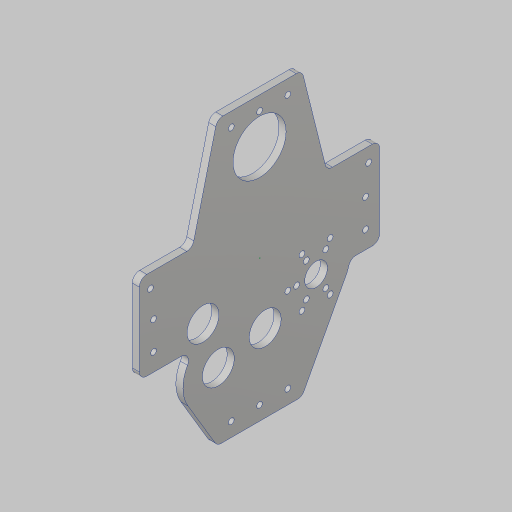
# Autodesk Inventor part: EL2-CGB-001
Saved by Autodesk Inventor 2023.5 (Build 275446000, 446)
## iProperties
Created: 2025-01-19
Part Number: EL2-CGB-001
Material: Aluminum 6061
Document SubType Name: Modeling
Designer: mavericks
Density: 2.7 g/cm^3
Appearance: Aluminum - Flat
Author: mavericks
Autodesk Inventor part; units mm, degrees
ref_plane "YZ Plane" through (0, 0, 0) normal (1, 0, 0) x (0, 1, 0)
ref_plane "XZ Plane" through (0, 0, 0) normal (0, 1, 0) x (-1, 0, 0)
ref_plane "XY Plane" through (0, 0, 0) normal (0, 0, 1) x (1, 0, 0)
sketch "Sketch1" plane through (0, 0, 0) normal (1, 0, 0) x (0, 1, 0)
  line L0 (127, 107.95) -> (-127, 107.95) construction
  line L1 (-127, 107.95) -> (-127, 82.55) construction
  line L2 (-127, 82.55) -> (127, 82.55) construction
  line L3 (127, 82.55) -> (127, 107.95) construction
  line L4 (-44.45, 128.7526) -> (-69.85, 128.7526) construction
  line L5 (-69.85, 128.7526) -> (-69.85, 79.4258) construction
  line L6 (-69.85, 79.4258) -> (-44.45, 79.4258) construction
  line L7 (-44.45, 79.4258) -> (-44.45, 128.7526) construction
  line L8 (69.85, 128.7526) -> (44.45, 128.7526) construction
  line L9 (44.45, 128.7526) -> (44.45, 79.4258) construction
  line L10 (44.45, 79.4258) -> (69.85, 79.4258) construction
  line L11 (69.85, 79.4258) -> (69.85, 128.7526) construction
  line L12 (44.45, 104.0892) -> (-44.45, 104.0892) construction
  line L13 (0, 0) -> (-27.2932, 0) construction
  line L14 (127, -107.95) -> (-127, -107.95) construction
  line L15 (-127, -107.95) -> (-127, -82.55) construction
  line L16 (-127, -82.55) -> (127, -82.55) construction
  line L17 (127, -82.55) -> (127, -107.95) construction
  line L18 (-44.45, -128.7526) -> (-69.85, -128.7526) construction
  line L19 (-69.85, -128.7526) -> (-69.85, -79.4258) construction
  line L20 (-69.85, -79.4258) -> (-44.45, -79.4258) construction
  line L21 (-44.45, -79.4258) -> (-44.45, -128.7526) construction
  line L22 (69.85, -128.7526) -> (44.45, -128.7526) construction
  line L23 (44.45, -128.7526) -> (44.45, -79.4258) construction
  line L24 (44.45, -79.4258) -> (69.85, -79.4258) construction
  line L25 (69.85, -79.4258) -> (69.85, -128.7526) construction
  line L26 (44.45, -104.0892) -> (-44.45, -104.0892) construction
  line L27 (127, 82.55) -> (101.6, 82.55) construction
  line L28 (101.6, 82.55) -> (101.6, -82.55) construction
  line L29 (101.6, -82.55) -> (127, -82.55) construction
  line L30 (127, -82.55) -> (127, 82.55) construction
  line L31 (-127, 82.55) -> (-101.6, 82.55) construction
  line L32 (-101.6, 82.55) -> (-101.6, -82.55) construction
  line L33 (-101.6, -82.55) -> (-127, -82.55) construction
  line L34 (-127, -82.55) -> (-127, 82.55) construction
  point P0 (0, 82.55)
  point P1 (0, 104.0892)
  point P2 (0, -82.55)
  point P3 (0, -104.0892)
  dimension "d0" = 254
  dimension "d1" = 25.4
  dimension "d2" = 82.55
  dimension "d3" = 25.4
  dimension "d4" = 49.3268
  dimension "d6" = 88.9
  dimension "d7" = 3.1242
  dimension "d8" = 25.4
  dimension "d9" = 25.4
  constraints: 70 end point, 16 symmetric about line, 12 parallel, 7 horizontal, 5 perpendicular, 4 midpoint, 2 vertical alignment, 1 horizontal alignment, 1 point on line
  measures "d0" distance of L2.end L1.end
  measures "d1" distance of L1.end L0.end
  measures "d2" vertical distance of L13.start L2.end
  measures "d3" distance of L6.end L5.end
  measures "d4" distance of L5.end L4.end
  measures "d6" distance of L4.start L8.end
  measures "d7" distance from line of L2 L6.end
  measures "d8" distance between parallel lines of L28 L30
  measures "d9" distance between parallel lines of L34 L32
sketch "Sketch2" plane through (0, 0, 0) normal (1, 0, 0) x (0, 1, 0)
  line L0 (-127, 107.95) -> (-127, 82.55) construction
  line L1 (44.45, 104.0892) -> (-44.45, 104.0892) construction
  line L2 (-127, 82.55) -> (127, 82.55) construction
  line L3 (127, 107.95) -> (-127, 107.95) construction
  line L4 (44.45, 79.4258) -> (69.85, 79.4258) construction
  line L5 (127, 82.55) -> (127, 107.95) construction
  line L6 (-69.85, 79.4258) -> (-44.45, 79.4258) construction
  line L7 (-44.45, 79.4258) -> (-44.45, 128.7526) construction
  line L8 (-69.85, 128.7526) -> (-69.85, 79.4258) construction
  line L9 (-44.45, 128.7526) -> (-69.85, 128.7526) construction
  line L10 (101.6, 82.55) -> (101.6, -82.55) construction
  line L11 (127, -82.55) -> (127, 82.55) construction
  line L12 (-127, -82.55) -> (127, -82.55) construction
  line L13 (127, -107.95) -> (-127, -107.95) construction
  line L14 (44.45, -104.0892) -> (-44.45, -104.0892) construction
  line L15 (-127, 82.55) -> (-101.6, 82.55) construction
  line L16 (-101.6, 82.55) -> (-101.6, -82.55) construction
  line L17 (-127, -82.55) -> (-127, 82.55) construction
  line L18 (-69.85, -79.4258) -> (-44.45, -79.4258) construction
  line L19 (-101.6, -82.55) -> (-127, -82.55) construction
  line L20 (-44.45, -79.4258) -> (-44.45, -128.7526) construction
  line L21 (-44.45, -128.7526) -> (-69.85, -128.7526) construction
  line L22 (-69.85, -128.7526) -> (-69.85, -79.4258) construction
  line L23 (-127, -107.95) -> (-127, -82.55) construction
  line L24 (44.45, -79.4258) -> (69.85, -79.4258) construction
  line L25 (44.45, -128.7526) -> (44.45, -79.4258) construction
  line L26 (101.6, -82.55) -> (127, -82.55) construction
  line L27 (69.85, -128.7526) -> (44.45, -128.7526) construction
  line L28 (69.85, -79.4258) -> (69.85, -128.7526) construction
  line L29 (127, -82.55) -> (127, -107.95) construction
  line L30 (69.85, 128.7526) -> (44.45, 128.7526) construction
  line L31 (44.45, 128.7526) -> (44.45, 79.4258) construction
  line L32 (69.85, 79.4258) -> (69.85, 128.7526) construction
  line L33 (127, 82.55) -> (101.6, 82.55) construction
  circle A0 centre (-38.1, -50.8) radius 7.62 construction
  circle A1 centre (-57.15, -5.08) radius 41.91 construction
  circle A2 centre (-57.15, -5.08) radius 11.43 construction
  circle A3 centre (-66.675, 37.0363) radius 31.75 construction
  circle A4 centre (-66.675, 37.0363) radius 15.24 construction
  circle A5 centre (-25.7473, 50.8) radius 27.94 construction
  circle A6 centre (-38.1, -50.8) radius 30.48 construction
  circle A7 centre (-38.1, -50.8) radius 10.16
  circle A8 centre (-57.15, -5.08) radius 14.2875
  circle A9 centre (-66.675, 37.0363) radius 14.2875
  circle A10 centre (-25.7473, 50.8) radius 14.2875
  circle A11 centre (-25.7473, 50.8) radius 20.6375 construction
  circle A12 centre (-66.675, 37.0363) radius 20.6375 construction
  circle A13 centre (-57.15, -5.08) radius 20.6375 construction
  circle A14 centre (-38.1, -50.8) radius 17.4625 construction
  circle A15 centre (-38.1, -50.8) radius 25.4 construction
  line L34 (-41.275, -131.9276) -> (-41.275, -76.2508) construction
  line L35 (-41.275, -76.2508) -> (-73.025, -76.2508) construction
  line L36 (-73.025, -76.2508) -> (-73.025, -131.9276) construction
  line L37 (-73.025, -131.9276) -> (-41.275, -131.9276) construction
  line L38 (-52.3959, -77.7195) -> (-127, -38.1)
  line L39 (-127, -38.1) -> (-127, 38.1)
  line L40 (-127, 38.1) -> (-41.275, 38.1) construction
  line L41 (-41.275, 38.1) -> (-41.275, 104.0892) construction
  arc A16 (-52.3959, -77.7195) -> (-41.275, -81.1142) centre (-38.1, -50.8) ccw
  circle A17 centre (86.4755, 0) radius 23.8125
  circle A18 centre (86.4755, 0) radius 33.3375 construction
  line L42 (37.9487, 60.325) -> (127, 38.1)
  line L43 (127, 38.1) -> (127, -38.1)
  line L44 (127, -38.1) -> (37.9487, -60.325)
  line L45 (37.9487, -60.325) -> (37.9487, -107.95)
  line L46 (37.9487, -107.95) -> (-41.275, -107.95)
  line L47 (-41.275, -107.95) -> (-41.275, -81.1142)
  line L48 (37.9487, 60.325) -> (37.9487, 107.95)
  line L49 (37.9487, 107.95) -> (-41.275, 107.95)
  arc A19 (-23.4758, 68.844) -> (-37.8063, 37.1865) centre (-25.7473, 50.8) ccw construction
  arc A20 (50.2903, -40.85) -> (93.2916, 54.1446) centre (86.4755, 0) ccw construction
  line L50 (-41.275, 107.95) -> (-41.275, 56.0863)
  line L51 (-82.9044, 64.325) -> (-127, 38.1)
  arc A21 (-41.275, 56.0863) -> (-82.9044, 64.325) centre (-66.675, 37.0363) ccw
  line L52 (93.2916, 54.1446) -> (-23.4758, 68.844) construction
  line L53 (50.2903, -40.85) -> (-37.8063, 37.1865) construction
  circle A22 centre (86.4755, 0) radius 11.1125 construction
  point P0 (25.2487, 98.0186)
  point P1 (0, 95.25)
  point P2 (25.2487, -98.0186)
  point P3 (0, -95.25)
  point P4 (-25.4, -95.25)
  point P5 (-25.4, 95.25)
  point P6 (127, -95.25)
  point P7 (127, 95.25)
  point P8 (0, -82.55)
  point P9 (-114.3, 25.4)
  point P10 (-114.3, 0)
  point P11 (-114.3, -25.4)
  point P12 (-101.6, 0)
  point P13 (-114.3, 82.55)
  point P14 (-38.1, -25.4)
  point P15 (-38.1, -33.3375)
  point P16 (-60.097, -38.1)
  point P17 (-53.223, -42.0688)
  point P18 (-60.097, -63.5)
  point P19 (-53.223, -59.5312)
  point P20 (-38.1, -76.2)
  point P21 (-38.1, -68.2625)
  point P22 (-16.103, -63.5)
  point P23 (-22.977, -59.5313)
  point P24 (-16.103, -38.1)
  point P25 (-22.977, -42.0688)
  point P26 (44.45, 104.0892)
  point P27 (-127, 0)
  point P28 (-127, 0)
  point P29 (101.6, 0)
  point P30 (114.3, 25.4)
  point P31 (114.3, 0)
  point P32 (114.3, -25.4)
  point P33 (114.3, 82.55)
  point P34 (127, 0)
  point P35 (-41.275, -76.8809)
  dimension "d33" = 34.925
  dimension "d34" = 50.8
  dimension "d10" = 15.24
  dimension "d11" = 83.82
  dimension "d12" = 22.86
  dimension "d13" = 63.5
  dimension "d14" = 30.48
  dimension "d15" = 55.88
  dimension "d16" = 60.96
  dimension "d19" = 63.5
  dimension "d23" = 20.32
  dimension "d24" = 28.575
  dimension "d26" = 25.4
  dimension "d27" = 25.4
  dimension "d28" = 25.4
  dimension "d29" = 25.4
  dimension "d30" = 6.35
  dimension "d31" = 6.35
  dimension "d32" = 6.35
  dimension "d37" = 360
  dimension "d41" = 3.175
  dimension "d42" = 76.2
  dimension "d60" = 101.7513
  dimension "d63" = 31.75
  dimension "d64" = 44.45
  dimension "d66" = 34.925
  dimension "d67" = 31.75
  dimension "d68" = 47.625
  dimension "d70" = 9.525
  dimension "d71" = 47.625
  dimension "d73" = 123.1853
  dimension "d74" = 12.7
  dimension "d75" = 36.3728
  dimension "d76" = 109.1438
  dimension "d78" = 9.9314
  dimension "d79" = 9.9314
  dimension "d133" = 204.1689
  dimension "d134" = 46.2281
  dimension "d135" = 117.689
  dimension "d141" = 22.225
  constraints: 40 end point, 21 centre point, 18 vertical alignment, 15 coincident, 12 point on circle, 11 horizontal alignment, 11 midpoint, 11 point on line, 9 tangent, 3 collinear, 2 equal radius, 2 perpendicular, 1 horizontal, 1 vertical, 20 other
  measures "d10" diameter of A0
  measures "d11" diameter of A1
  measures "d12" diameter of A2
  measures "d13" diameter of A3
  measures "d14" diameter of A4
  measures "d15" diameter of A5
  measures "d16" diameter of A6
  measures "d19" distance from line of L16 A0.centre
  measures "d23" diameter of A7
  measures "d24" diameter of A8
  measures "d26" distance of point (-25.4, 95.25) point (0, 95.25)
  measures "d27" distance of point (25.249, 98.019) point (0, 95.25)
  measures "d28" distance of point (-114.3, 0) point (-114.3, 25.4)
  measures "d29" distance of point (-114.3, 0) point (-114.3, -25.4)
  measures "d30" radial gap between concentric circles of A10 A11
  measures "d31" radial gap between concentric circles of A9 A12
  measures "d32" radial gap between concentric circles of A8 A13
  measures "d41" distance between parallel lines of L20 L34
  measures "d42" distance of L38.end L39.end
  measures "d60" distance from line of L5 point (25.249, 98.019)
  measures "d63" distance from line of L12 A0.centre
  measures "d64" distance from line of L16 A1.centre
  measures "d66" distance from line of L16 A3.centre
  measures "d67" distance from line of L2 A5.centre
  measures "d68" diameter of A17
  measures "d70" radial gap between concentric circles of A17 A18
  measures "d71" distance of L42.start L48.end
  measures "d73" distance of A17.centre A5.centre
  measures "d74" horizontal distance of point (25.249, 98.019) L48.end
  measures "d75" diameter of A19
  measures "d76" diameter of A20
  measures "d78" distance from line of point (25.249, 98.019) L3
  measures "d79" distance from line of L13 point (25.249, -98.019)
  measures "d135" distance of L52.start L52.end
  measures "d141" diameter of A22
extrude "Extrusion1" add sketch "Sketch2" along normal blind 6.35
hole "Mount Holes" at (0, -101.6, 82.55) at (0, -127, 107.95) at (0, -69.85, 79.4258) at (0, 44.45, -79.4258) at (0, 69.85, -79.4258) at (0, 44.45, -128.7526) at (0, 44.45, 128.7526) at (0, 25.2487, 98.0186) at (0, 0, 95.25) at (0, 25.2487, -98.0186) at (0, 0, -95.25) at (0, -25.4, -95.25) at (0, -25.4, 95.25) at (0, -114.3, 25.4) at (0, -114.3, 0) at (0, -114.3, -25.4) at (0, 114.3, 25.4) at (0, 114.3, 0) at (0, 114.3, -25.4) direction (1, 0, 0) diameter 5.1054 end through all clearance for "Flat Head Machine Screw (82)" size "#10" standard "Ansi Unified Screw Threads"
hole "Motor Mount Holes" at (0, -38.1, -33.3375) at (0, -60.097, -38.1) at (0, -53.223, -42.0688) at (0, -60.097, -63.5) at (0, -53.223, -59.5312) at (0, -16.103, -63.5) at (0, -22.977, -59.5313) at (0, -16.103, -38.1) at (0, -22.977, -42.0688) at (0, -38.1, -25.4) direction (1, 0, 0) diameter 5.1054 end through all clearance for "Flat Head Machine Screw (82)" size "#10" standard "Ansi Unified Screw Threads"
sketch "Sketch3" plane through (6.35, 0, 0) normal (1, 0, 0) x (0, 0, -1)
  point P0 (0, 0)
fillet "Fillet1" radius 6.604 12 edges at (3.175, -41.275, 107.95) (3.175, -127, 38.1) (3.175, -127, -38.1) (3.175, -41.275, -81.1142) (3.175, -41.275, -107.95) (3.175, 37.9487, -107.95) (3.175, 37.9487, -60.325) (3.175, 127, -38.1) (3.175, 127, 38.1) (3.175, 37.9487, 60.325) (3.175, 37.9487, 107.95) (3.175, -41.275, 56.0863)
sketch "Sketch4" plane through (6.35, 0, 0) normal (1, 0, 0) x (0, 0, -1)
  arc A0 (-107.95, -34.671) -> (-101.346, -41.275) centre (-101.346, -34.671) ccw construction
  line L0 (-107.95, -34.671) -> (-107.95, 31.3447) construction
  arc A1 (-101.346, 37.9487) -> (-107.95, 31.3447) centre (-101.346, 31.3447) ccw construction
  line L1 (-101.346, 37.9487) -> (-65.4834, 37.9487) construction
  arc A2 (-65.4834, 37.9487) -> (-59.0759, 42.9535) centre (-65.2807, 44.5527) ccw construction
  line L2 (-58.8844, 42.8978) -> (-39.4851, 109.5417) construction
  arc A3 (-33.1443, 114.3) -> (-39.4851, 109.5417) centre (-33.1443, 107.696) ccw construction
  line L3 (-33.1443, 114.3) -> (33.1443, 114.3) construction
  arc A4 (39.4851, 109.5417) -> (33.1443, 114.3) centre (33.1443, 107.696) ccw construction
  line L4 (39.4851, 109.5417) -> (58.9399, 42.7069) construction
  arc A5 (58.9399, 42.7069) -> (65.2807, 37.9487) centre (65.2807, 44.5527) ccw construction
  line L5 (65.2807, 37.9487) -> (101.346, 37.9487) construction
  arc A6 (107.95, 31.3447) -> (101.346, 37.9487) centre (101.346, 31.3447) ccw construction
  line L6 (107.95, 31.3447) -> (107.95, -34.671) construction
  arc A7 (101.346, -41.275) -> (107.95, -34.671) centre (101.346, -34.671) ccw construction
  line L7 (101.346, -41.275) -> (76.8809, -41.275) construction
  line L8 (76.8809, -41.275) -> (39.9622, -110.7934) construction
  arc A8 (34.1297, -114.3) -> (39.9622, -110.7934) centre (34.1297, -107.696) ccw construction
  line L9 (34.1297, -114.3) -> (-34.3439, -114.3) construction
  arc A9 (-40.02, -111.0717) -> (-34.3439, -114.3) centre (-34.3439, -107.696) ccw construction
  line L10 (-40.02, -111.0717) -> (-64.325, -70.2044) construction
  arc A10 (-68.3827, -48.9286) -> (-64.325, -70.2044) centre (-37.0363, -53.975) ccw construction
  arc A11 (-68.3827, -48.9286) -> (-74.9028, -41.275) centre (-74.9028, -47.879) ccw construction
  line L11 (-74.9028, -41.275) -> (-101.346, -41.275) construction
  circle A12 centre (38.1, -3.403) radius 2.5527 construction
  circle A13 centre (63.5, -3.403) radius 2.5527 construction
  circle A14 centre (63.5, -47.397) radius 2.5527 construction
  circle A15 centre (38.1, -47.397) radius 2.5527 construction
  circle A16 centre (33.3375, -25.4) radius 2.5527 construction
  circle A17 centre (42.0688, -40.523) radius 2.5527 construction
  circle A18 centre (59.5312, -40.523) radius 2.5527 construction
  circle A19 centre (59.5313, -10.277) radius 2.5527 construction
  circle A20 centre (42.0688, -10.277) radius 2.5527 construction
  circle A21 centre (0, 101.6) radius 2.5527 construction
  circle A22 centre (25.4, -101.6) radius 2.5527 construction
  circle A23 centre (-25.4, -101.6) radius 2.5527 construction
  circle A24 centre (95.25, -25.4) radius 2.5527 construction
  circle A25 centre (98.0186, 25.2487) radius 2.5527 construction
  circle A26 centre (-98.0186, 25.2487) radius 2.5527 construction
  circle A27 centre (-95.25, 0) radius 2.5527 construction
  circle A28 centre (95.25, 0) radius 2.5527 construction
  circle A29 centre (-95.25, -25.4) radius 2.5527 construction
  circle A30 centre (0, -101.6) radius 2.5527 construction
  circle A31 centre (-25.4, 101.6) radius 2.5527 construction
  circle A32 centre (25.4, 101.6) radius 2.5527 construction
  circle A33 centre (0, 58.3056) radius 23.8125 construction
  circle A34 centre (-50.8, -13.0473) radius 14.2875 construction
  circle A35 centre (-37.0363, -53.975) radius 14.2875 construction
  circle A36 centre (5.08, -44.45) radius 14.2875 construction
  circle A37 centre (50.8, -25.4) radius 10.16 construction
  circle A38 centre (0, 58.3056) radius 30.1625 construction
  circle A39 centre (-50.8, -13.0473) radius 20.6375 construction
  circle A40 centre (-37.0363, -53.975) radius 20.6375 construction
  circle A41 centre (5.08, -44.45) radius 20.6375 construction
  circle A42 centre (38.1, -3.403) radius 8.9027 construction
  circle A43 centre (63.5, -3.403) radius 8.9027 construction
  line L12 (0, 58.3056) -> (-50.8, -13.0473) construction
  circle A44 centre (63.5, -16.103) radius 2.5527 construction
  line L13 (0, 58.3056) -> (69.8474, -9.5713) construction
  line L14 (0, 58.3056) -> (5.08, -44.45) construction
  line L15 (-47.1323, -13.3701) -> (0.4406, 53.4502) construction
  line L16 (0.4406, 53.4502) -> (74.8023, -18.8136) construction
  line L17 (-52.3052, -9.6872) -> (-0.4406, 63.1611) construction
  line L18 (-0.4406, 63.1611) -> (79.2277, -14.2597) construction
  line L19 (8.3838, -46.9773) -> (3.5692, 50.4098) construction
  line L20 (3.5692, 50.4098) -> (74.8023, -18.8136) construction
  line L21 (2.0416, -47.2908) -> (-3.5692, 66.2014) construction
  line L22 (-3.5692, 66.2014) -> (79.2277, -14.2597) construction
  line L23 (-65.2807, 31.5987) -> (-101.346, 31.5987) construction
  arc A45 (-101.346, 31.5987) -> (-101.6, 31.3447) centre (-101.346, 31.3447) ccw construction
  line L24 (-101.6, 31.3447) -> (-101.6, -34.671) construction
  arc A46 (-101.6, -34.671) -> (-101.346, -34.925) centre (-101.346, -34.671) ccw construction
  line L25 (-101.346, -34.925) -> (-74.9028, -34.925) construction
  arc A47 (-62.1135, -49.9379) -> (-74.9028, -34.925) centre (-74.9028, -47.879) ccw construction
  arc A48 (-62.1135, -49.9379) -> (-58.8673, -66.9585) centre (-37.0363, -53.975) ccw construction
  line L26 (-58.8673, -66.9585) -> (-34.5622, -107.8258) construction
  arc A49 (-34.5622, -107.8258) -> (-34.3439, -107.95) centre (-34.3439, -107.696) ccw construction
  line L27 (-34.3439, -107.95) -> (34.1297, -107.95) construction
  arc A50 (34.1297, -107.95) -> (34.354, -107.8151) centre (34.1297, -107.696) ccw construction
  line L28 (34.354, -107.8151) -> (71.2726, -38.2967) construction
  arc A51 (71.2726, -38.2967) -> (62.2649, -29.6267) centre (44.45, -57.15) ccw construction
  arc A52 (58.1608, -34.925) -> (62.2649, -29.6267) centre (80.3564, -47.879) ccw construction
  line L29 (58.1608, -34.925) -> (101.346, -34.925) construction
  arc A53 (101.346, -34.925) -> (101.0948, -34.7088) centre (101.346, -34.671) ccw construction
  line L30 (101.6, -34.925) -> (101.6, 31.3447) construction
  arc A54 (101.6, 31.3447) -> (101.346, 31.5987) centre (101.346, 31.3447) ccw construction
  line L31 (101.346, 31.5987) -> (65.2807, 31.5987) construction
  arc A55 (52.843, 40.9322) -> (65.2807, 31.5987) centre (65.2807, 44.5527) ccw construction
  line L32 (52.843, 40.9322) -> (33.3881, 107.767) construction
  arc A56 (33.3881, 107.767) -> (33.1443, 107.95) centre (33.1443, 107.696) ccw construction
  line L33 (33.1443, 107.95) -> (-33.1443, 107.95) construction
  arc A57 (-33.1443, 107.95) -> (-33.3881, 107.767) centre (-33.1443, 107.696) ccw construction
  line L34 (-33.3881, 107.767) -> (-52.843, 40.9322) construction
  arc A58 (-65.2807, 31.5987) -> (-52.843, 40.9322) centre (-65.2807, 44.5527) ccw construction
  circle A59 centre (0, -114.3) radius 2.5527 construction
  circle A60 centre (38.1, -60.097) radius 2.5527 construction
  circle A61 centre (38.1, -47.397) radius 8.9027 construction
  circle A62 centre (-25.4, -101.6) radius 8.9027 construction
  circle A63 centre (25.4, -101.6) radius 8.9027 construction
  line L35 (-14.81, 32.0294) -> (-36.3867, 1.723)
  line L36 (19.2982, 35.1246) -> (55.3225, 0.1166)
  line L37 (-31.239, -6.4691) -> (-25.4065, -23.8125)
  line L38 (40.9805, 5.0209) -> (55.3225, 0.1166)
  line L39 (-25.4065, -23.8125) -> (0.8809, -23.8125)
  arc A64 (-31.239, -6.4691) -> (-36.3867, 1.723) centre (-50.8, -13.0473) ccw
  arc A65 (40.9805, 5.0209) -> (32.5805, 3.5823) centre (38.1, -3.403) ccw
  arc A66 (-14.81, 32.0294) -> (19.2982, 35.1246) centre (0, 58.3056) ccw
  line L40 (6.8879, -16.719) -> (4.6522, 28.5041)
  line L41 (-1.6901, 28.1905) -> (0.8809, -23.8125)
  line L42 (6.8879, -16.719) -> (32.5805, 3.5823)
  line L43 (59.9983, 0) -> (57.5056, 34.1915) construction
  circle A67 centre (95.25, -25.4) radius 2.5527 construction
  line L44 (59.9983, 0) -> (95.25, 0) construction
  line L45 (60.8203, 32.3908) -> (62.9502, 3.175) construction
  line L46 (62.9502, 3.175) -> (95.5186, 3.175) construction
  line L47 (54.0356, 38.122) -> (57.0463, -3.175) construction
  line L48 (57.0463, -3.175) -> (95.25, -3.175) construction
  circle A68 centre (95.25, -25.4) radius 8.9027 construction
  circle A69 centre (95.25, 0) radius 8.9027 construction
  circle A70 centre (98.0186, 25.2487) radius 8.9027 construction
  circle A71 centre (98.0186, 25.2487) radius 2.5527 construction
  arc A72 (91.7788, 31.5987) -> (101.6, 17.0981) centre (98.0186, 25.2487) ccw
  circle A73 centre (95.25, 0) radius 2.5527 construction
  arc A74 (101.6, 6.2398) -> (86.9327, 3.175) centre (95.25, 0) ccw
  arc A75 (86.9327, -3.175) -> (101.6, -6.2398) centre (95.25, 0) ccw
  arc A76 (101.6, -19.1602) -> (88.9, -31.6398) centre (95.25, -25.4) ccw
  line L49 (61.9926, -15.9214) -> (60.0394, -32.1415) construction
  line L50 (63.6988, -28.3093) -> (66.8402, -2.2217) construction
  line L51 (66.8402, -2.2217) -> (-3.5692, 66.2014) construction
  line L52 (-3.5692, 66.2014) -> (2.0416, -47.2908) construction
  line L53 (57.7912, -24.2546) -> (60.1598, -4.5842) construction
  line L54 (60.1598, -4.5842) -> (3.5692, 50.4098) construction
  line L55 (3.5692, 50.4098) -> (8.3838, -46.9773) construction
  line L56 (60.8203, 32.3908) -> (62.9502, 3.175)
  line L57 (62.9502, 3.175) -> (86.9327, 3.175)
  line L58 (86.9327, -3.175) -> (67.8212, -3.175)
  line L59 (67.8212, -3.175) -> (59.748, 4.6705)
  arc A77 (65.6579, -12.0402) -> (59.748, 4.6705) centre (63.5, -3.403) ccw
  arc A78 (58.1608, -34.925) -> (63.6988, -28.3093) centre (80.3564, -47.879) ccw
  line L60 (58.1608, -34.925) -> (88.9, -34.925)
  line L61 (63.6988, -28.3093) -> (65.6579, -12.0402)
  line L62 (91.7788, 31.5987) -> (65.2807, 31.5987)
  arc A79 (60.8203, 32.3908) -> (65.2807, 31.5987) centre (65.2807, 44.5527) ccw
  line L63 (101.6, 17.0981) -> (101.6, 6.2398)
  line L64 (29.4865, 51.9556) -> (49.6342, 51.9556)
  arc A80 (23.7236, 39.6786) -> (29.4865, 51.9556) centre (0, 58.3056) ccw
  arc A81 (52.843, 40.9322) -> (54.0356, 38.122) centre (65.2807, 44.5527) ccw
  line L65 (49.6342, 51.9556) -> (52.843, 40.9322)
  line L66 (54.0356, 38.122) -> (56.2247, 8.0943)
  line L67 (56.2247, 8.0943) -> (23.7236, 39.6786)
  line L68 (-29.4865, 51.9556) -> (-49.6342, 51.9556)
  line L69 (-50.8, -13.0473) -> (-57.5056, 34.1915) construction
  line L70 (-47.6565, -12.6011) -> (-54.7072, 37.0689) construction
  line L71 (-53.9435, -13.4936) -> (-60.1282, 30.0756) construction
  circle A82 centre (-95.25, 0) radius 8.9027 construction
  circle A83 centre (-98.0186, 25.2487) radius 8.9027 construction
  circle A84 centre (-95.25, -25.4) radius 8.9027 construction
  circle A85 centre (-95.25, 0) radius 2.5527 construction
  line L72 (-95.25, 0) -> (-66.7898, 0) construction
  line L73 (-95.25, 3.175) -> (-63.5571, 3.175) construction
  line L74 (-95.25, -3.175) -> (-69.223, -3.175) construction
  line L75 (-65.2807, 31.5987) -> (-91.7788, 31.5987)
  line L76 (-101.6, 17.0981) -> (-101.6, 6.2398)
  line L77 (-101.6, -6.2398) -> (-101.6, -19.1602)
  line L78 (-88.9, -34.925) -> (-74.9028, -34.925)
  line L79 (-62.1135, -49.9379) -> (-57.2751, -49.9379)
  line L80 (-86.9327, 3.175) -> (-63.5571, 3.175)
  line L81 (-68.923, -3.175) -> (-86.9327, -3.175)
  line L82 (-60.4755, 32.5229) -> (-56.8094, 6.6959)
  line L83 (-50.5224, 7.5883) -> (-54.7072, 37.0689)
  line L84 (-41.5596, 5.4059) -> (-19.9829, 35.7123)
  circle A86 centre (-98.0186, 25.2487) radius 2.5527 construction
  arc A87 (-101.6, 17.0981) -> (-91.7788, 31.5987) centre (-98.0186, 25.2487) ccw
  arc A88 (-86.9327, 3.175) -> (-101.6, 6.2398) centre (-95.25, 0) ccw
  arc A89 (-101.6, -6.2398) -> (-86.9327, -3.175) centre (-95.25, 0) ccw
  arc A90 (-88.9, -31.6398) -> (-101.6, -19.1602) centre (-95.25, -25.4) ccw
  arc A91 (-62.1135, -49.9379) -> (-74.9028, -34.925) centre (-74.9028, -47.879) ccw
  arc A92 (-49.7363, -37.708) -> (-57.2751, -49.9379) centre (-37.0363, -53.975) ccw
  line L85 (-49.7363, -37.708) -> (-49.7363, -33.6574)
  arc A93 (-68.923, -3.175) -> (-49.7363, -33.6574) centre (-50.8, -13.0473) ccw
  arc A94 (-56.8094, 6.6959) -> (-63.5571, 3.175) centre (-50.8, -13.0473) ccw
  arc A95 (-65.4834, 37.9487) -> (-59.0759, 42.9535) centre (-65.4834, 44.5527) ccw construction
  arc A96 (-65.2807, 31.5987) -> (-60.4755, 32.5229) centre (-65.2807, 44.5527) ccw
  arc A97 (-29.4865, 51.9556) -> (-19.9829, 35.7123) centre (0, 58.3056) ccw
  line L86 (-49.6342, 51.9556) -> (-52.843, 40.9322)
  arc A98 (-54.7072, 37.0689) -> (-52.843, 40.9322) centre (-65.2807, 44.5527) ccw
  line L87 (-43.3863, -73.6113) -> (-49.5945, -82.55)
  line L88 (-25.4, -92.6973) -> (25.4, -92.6973)
  line L89 (25.4, -92.6973) -> (29.2279, -46.6594)
  line L90 (29.2325, -46.6056) -> (25.6358, -46.2846)
  line L91 (-11.187, -57.15) -> (-16.6445, -57.15)
  line L92 (-49.5945, -82.55) -> (-34.4884, -107.95)
  line L93 (-34.4884, -107.95) -> (-31.6398, -107.95)
  arc A99 (-43.3863, -73.6113) -> (-16.6445, -57.15) centre (-37.0363, -53.975) ccw
  arc A100 (-11.187, -57.15) -> (25.6358, -46.2846) centre (5.08, -44.45) ccw
  arc A101 (29.2325, -46.6056) -> (29.2279, -46.6594) centre (38.1, -47.397) ccw
  circle A102 centre (-25.4, -114.3) radius 2.5527 construction
  arc A103 (-25.4, -92.6973) -> (-31.6398, -107.95) centre (-25.4, -101.6) ccw
  arc A104 (-41.5596, 5.4059) -> (-50.5224, 7.5883) centre (-50.8, -13.0473) ccw
  line L94 (101.6, -19.1602) -> (101.6, -6.2398)
  line L95 (-88.9, -31.6398) -> (-88.9, -34.925)
  line L96 (88.9, -34.925) -> (88.9, -31.6398)
  circle A105 centre (25.4, -25.4) radius 2.5527 projected
  point P0 (0, 0)
  point P1 (60.0394, -32.1415)
  point P2 (31.75, 27.4513)
  point P3 (-49.7363, -35.6827)
  point P4 (-42.0415, -95.25)
  point P5 (-51.5708, -29.9236)
  point P6 (30.5287, -26.3344)
  point P7 (-101.6, 6.2398)
  point P8 (-88.9, -33.2824)
  point P9 (88.9, -33.2824)
  point P10 (72.3998, -3.175)
  point P11 (86.685, -22.9712)
  dimension "d80" = 6.35
  dimension "d81" = 6.35
  dimension "d82" = 6.35
  dimension "d83" = 6.35
  dimension "d84" = 6.35
  dimension "d85" = 6.35
  dimension "d86" = 3.175
  dimension "d87" = 3.175
  dimension "d88" = 3.175
  dimension "d89" = 3.175
  dimension "d90" = 6.35
  dimension "d91" = 6.35
  dimension "d94" = 6.35
  dimension "d95" = 6.35
  dimension "d96" = 3.175
  dimension "d97" = 3.175
  dimension "d98" = 6.35
  dimension "d99" = 6.35
  dimension "d100" = 6.35
  dimension "d101" = 3.175
  dimension "d102" = 3.175
  dimension "d103" = 3.175
  dimension "d104" = 3.175
  dimension "d105" = 3.175
  dimension "d106" = 6.35
  dimension "d107" = 3.175
  dimension "d108" = 3.175
  dimension "d109" = 6.35
  dimension "d110" = 6.35
  dimension "d111" = 6.35
  dimension "d112" = 3.175
  dimension "d113" = 3.175
  dimension "d114" = 12.7
  dimension "d115" = 6.35
  dimension "d116" = 31.75
  dimension "d117" = 12.7
  dimension "d121" = 12.7
  dimension "d122" = 12.7
  constraints: 169 end point, 129 point on circle, 53 centre point, 39 point on line, 23 coincident, 9 horizontal, 8 collinear, 8 tangent, 5 parallel, 4 horizontal alignment, 4 midpoint, 4 vertical alignment, 3 vertical, 2 concentric, 2 line through centre, 56 other
  measures "d80" radial gap between concentric circles of A33 A38
  measures "d82" radial gap between concentric circles of A35 A40
  measures "d83" radial gap between concentric circles of A36 A41
  measures "d84" radial gap between concentric circles of A12 A42
  measures "d85" radial gap between concentric circles of A13 A43
  measures "d86" distance between parallel lines of L12 L15
  measures "d87" distance between parallel lines of L12 L17
  measures "d88" distance between parallel lines of L14 L19
  measures "d89" distance between parallel lines of L14 L21
  measures "d90" distance between parallel lines of L1 L23
  measures "d91" radial gap between concentric circles of A15 A61
  measures "d94" radial gap between concentric circles of A23 A62
  measures "d96" distance between parallel lines of L43 L45
  measures "d97" distance between parallel lines of L43 L47
  measures "d99" radial gap between concentric circles of A28 A69
  measures "d100" radial gap between concentric circles of A25 A70
  measures "d101" distance between parallel lines of L49 L50
  measures "d102" distance between parallel lines of L49 L53
  measures "d103" distance between parallel lines of L44 L46
  measures "d104" distance between parallel lines of L44 L48
  measures "d105" distance from line of point (31.75, 27.451) L51
  measures "d106" distance from line of L12.start L64
  measures "d107" distance between parallel lines of L69 L70
  measures "d108" distance between parallel lines of L69 L71
  measures "d109" radial gap between concentric circles of A27 A82
  measures "d110" radial gap between concentric circles of A26 A83
  measures "d112" distance between parallel lines of L72 L73
  measures "d113" distance between parallel lines of L72 L74
  measures "d114" horizontal distance of A92.centre point (-49.736, -35.683)
  measures "d115" horizontal distance of L87.start A10.centre
  measures "d116" distance from line of L9 L87.end
  measures "d117" distance from line of L14.end L91
  measures "d121" distance from line of L24 point (-88.9, -33.282)
  measures "d122" distance from line of L30 point (88.9, -33.282)
body "Solid1"
